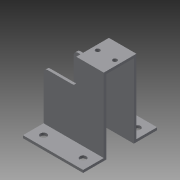
# Autodesk Inventor part: Autonomous - Ultrasonic Servo Mount
Saved by Autodesk Inventor 2014 (Build 180170000, 170)
## iProperties
Created: 2015-04-23
Part Number: Autonomous - Ultrasonic Servo Mount
Material: Generic
Document SubType Name: Modeling
Designer: WillHuie
Density: 1 g/cm^3
Appearance: Default
Author: WillHuie
Autodesk Inventor part; units mm, degrees
ref_plane "YZ Plane" through (0, 0, 0) normal (1, 0, 0) x (0, 1, 0)
ref_plane "XZ Plane" through (0, 0, 0) normal (0, 1, 0) x (-1, 0, 0)
ref_plane "XY Plane" through (0, 0, 0) normal (0, 0, 1) x (1, 0, 0)
sketch "Sketch1" plane through (0, 0, 0) normal (0, 1, 0) x (-1, 0, 0)
  line L0 (20.32, 10.16) -> (-20.32, 10.16)
  line L1 (-20.32, 10.16) -> (-20.32, -10.16)
  line L2 (-20.32, -10.16) -> (20.32, -10.16)
  line L3 (20.32, -10.16) -> (20.32, 10.16)
  line L4 (22.225, 12.065) -> (-22.225, 12.065)
  line L5 (-22.225, 12.065) -> (-22.225, -12.065)
  line L6 (-22.225, -12.065) -> (22.225, -12.065)
  line L7 (22.225, -12.065) -> (22.225, 12.065)
  point P0 (0, 0)
  dimension "d0" = 40.64
  dimension "d1" = 20.32
  dimension "d2" = 40.64
  dimension "d3" = 44.45
  dimension "d4" = 24.13
  dimension "d5" = 44.45
  constraints: 16 end point, 3 perpendicular, 2 parallel, 1 horizontal
  measures "d0" distance of L0.start L0.end
  measures "d1" distance of L0.end L1.end
  measures "d2" distance of L1.end L2.end
  measures "d3" distance of L4.start L4.end
  measures "d4" distance of L4.end L5.end
  measures "d5" distance of L5.end L6.end
extrude "Extrusion1" add sketch "Sketch1" along normal blind 56.515
sketch "Sketch2" plane through (-20.32, 0, -10.16) normal (1, 0, 0) x (0, 0, -1)
  line L0 (0, 0) -> (-20.32, 0) projected
  line L1 (0, 0) -> (0, 56.515) projected
  line L2 (-20.32, 56.515) -> (0, 56.515) projected
  line L3 (-20.32, 0) -> (-20.32, 56.515) projected
  point P0 (-10.16, 0)
extrude "Extrusion2" cut sketch "Sketch2" against normal blind 56.515
sketch "Sketch3" plane through (20.32, 0, 10.16) normal (-1, 0, 0) x (0, 0, 1)
  line L0 (0, 0) -> (-20.32, 0) projected
  line L1 (0, 0) -> (0, 56.515) projected
  line L2 (-20.32, 56.515) -> (0, 56.515) projected
  line L3 (-20.32, 0) -> (-20.32, 56.515) projected
  point P0 (-10.16, 0)
extrude "Extrusion3" cut sketch "Sketch3" against normal blind 56.515
sketch "Sketch4" plane through (22.225, 0, 10.16) normal (0, 0, -1) x (-1, 0, 0)
  line L0 (44.45, 56.515) -> (44.45, 0) projected
  line L1 (0, 56.515) -> (44.45, 56.515) projected
  line L2 (0, 0) -> (0, 56.515) projected
  line L3 (44.45, 54.61) -> (0, 54.61)
  point P0 (22.225, 0)
  constraints: 2 end point, 2 point on line, 1 perpendicular
extrude "Extrusion4" add sketch "Sketch4" along normal blind 20.32
sketch "Sketch5" plane through (-22.225, 0, 12.065) normal (0, 0, 1) x (1, 0, 0)
  line L0 (0, 0) -> (44.45, 0) projected
  line L1 (44.45, 0) -> (44.45, 56.515) projected
  line L2 (0, 0) -> (0, 56.515) projected
  line L3 (44.45, 1.905) -> (0, 1.905)
  point P0 (22.225, 0)
  constraints: 2 end point, 2 point on line, 1 perpendicular
extrude "Extrusion5" add sketch "Sketch5" along normal blind 15.24
sketch "Sketch6" plane through (22.225, 0, -12.065) normal (0, 0, -1) x (-1, 0, 0)
  line L0 (0, 0) -> (44.45, 0) projected
  line L1 (44.45, 0) -> (44.45, 56.515) projected
  line L2 (0, 0) -> (0, 56.515) projected
  line L3 (44.45, 1.905) -> (0, 1.905)
  point P0 (22.225, 0)
  constraints: 2 end point, 2 point on line, 1 perpendicular
extrude "Extrusion6" add sketch "Sketch6" along normal blind 15.24
sketch "Sketch7" plane through (0, 56.515, 0) normal (0, 1, 0) x (1, 0, 0)
  circle A0 centre (18.415, 0) radius 1.5875
  circle A1 centre (5.715, 0) radius 1.5875
  circle A2 centre (-12.065, 0) radius 3.175
  point P0 (0, 0)
  dimension "d18" = 3.175
  dimension "d19" = 3.175
  dimension "d20" = 6.35
  constraints: 3 centre point
  measures "d18" diameter of A0
  measures "d19" diameter of A1
  measures "d20" diameter of A2
extrude "Extrusion7" cut sketch "Sketch7" against normal blind 15.24
sketch "Sketch8" plane through (-22.225, 1.905, 12.065) normal (0, 1, 0) x (1, 0, 0)
  circle A0 centre (7.62, -7.62) radius 2.3495
  circle A1 centre (36.83, -7.62) radius 2.3495
  point P0 (22.225, 12.065)
  dimension "d23" = 4.699
  dimension "d24" = 4.699
  constraints: 2 centre point
  measures "d23" diameter of A0
  measures "d24" diameter of A1
extrude "Extrusion8" cut sketch "Sketch8" against normal blind 15.24
sketch "Sketch9" plane through (-22.225, 1.905, -12.065) normal (0, 1, 0) x (1, 0, 0)
  circle A0 centre (7.62, 7.62) radius 2.3495
  circle A1 centre (37.465, 7.62) radius 2.3495
  point P0 (22.225, -12.065)
  dimension "d27" = 4.699
  dimension "d28" = 4.699
  constraints: 2 centre point
  measures "d27" diameter of A0
  measures "d28" diameter of A1
extrude "Extrusion9" cut sketch "Sketch9" against normal blind 15.24
sketch "Sketch10" plane through (0, 56.515, 0) normal (0, 1, 0) x (1, 0, 0)
  circle A0 centre (-12.065, 0) radius 3.175 projected
  line L0 (-22.225, 12.065) -> (-22.225, -12.065) projected
  line L1 (-22.225, -12.065) -> (22.225, -12.065) projected
  line L2 (22.225, 12.065) -> (-22.225, 12.065) projected
  line L3 (1.905, 12.065) -> (1.905, -12.065)
  point P0 (0, 0)
  constraints: 2 end point, 2 point on line, 1 perpendicular
extrude "Extrusion10" cut sketch "Sketch10" against normal blind 19.05
fillet "Fillet1" radius 3.175 1 edges at (-22.225, 37.465, 11.1125)
fillet "Fillet2" radius 3.175 1 edges at (-22.225, 37.465, -11.1125)
fillet "Fillet3" radius 3.175 1 edges at (1.905, 37.465, 11.1125)
fillet "Fillet4" radius 3.175 1 edges at (1.905, 37.465, -11.1125)
body "Solid1"
